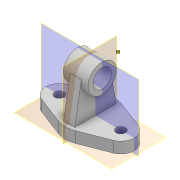
# Autodesk Inventor part: 6.2_DATE11_1
Saved by Autodesk Inventor 2017 (Build 210142000, 142)
## iProperties
Created: 2018-11-01
Part Number: 6.2_DATE11_1
Material: Generic
Document SubType Name: Modeling
Designer: jacob
Density: 1 g/cm^3
Appearance: Default
Mass: 222.641 g
Surface Area: 395.923 cm^2
Volume: 222.641 cm^3
Author: jacob
Autodesk Inventor part; units mm, degrees
sketch "Sketch1" plane through (0, 0, 0) normal (0, 0, 1) x (1, 0, 0)
  circle A0 centre (-49.8513, 0) radius 7.5
  circle A1 centre (50.2519, 0) radius 7.5
  line L0 (-57.7949, 20.5158) -> (-14.443, 37.3015)
  arc A2 (-57.7949, 20.5158) -> (-57.7949, -20.5158) centre (-49.8513, 0) ccw
  arc A3 (58.1322, -20.5402) -> (58.1322, 20.5402) centre (50.2519, 0) ccw
  line L1 (14.3278, 37.3459) -> (58.1322, 20.5402)
  line L2 (58.1322, -20.5402) -> (14.3278, -37.3459)
  line L3 (-57.7949, -20.5158) -> (-14.443, -37.3015)
  arc A4 (-14.443, -37.3015) -> (14.3278, -37.3459) centre (0, 0) ccw
  arc A5 (14.3278, 37.3459) -> (-14.443, 37.3015) centre (0, 0) ccw
  dimension "d19" = 15
  dimension "d20" = 15
  dimension "d45" = 44
  dimension "d46" = 44
  dimension "d47" = 0
  dimension "d48" = 0
  constraints: 8 end point, 8 point on circle, 8 tangent, 6 centre point, 3 coincident
  measures "d19" diameter of A0
  measures "d20" diameter of A1
  measures "d45" diameter of A2
  measures "d46" diameter of A3
  measures "d47" vertical distance of point (0, 0) A0.centre
  measures "d48" vertical distance of point (0, 0) A1.centre
sketch "Sketch2" plane through (0, 0, 0) normal (1, 0, 0) x (0, 1, 0)
  line L0 (-20.5849, 0) -> (20.5849, 0) projected
  line L1 (20.5849, 0) -> (20.5849, 18) projected
  line L2 (-20.5849, 18) -> (-20.5849, 18) projected
  line L3 (-20.5849, 0) -> (-20.5849, 18) projected
  line L4 (-20.5849, 18) -> (-20.5849, 18) projected
  line L5 (-33.5, 18) -> (33.5, 18)
  line L6 (33.5, 18) -> (22.6557, 79.9649)
  line L7 (-22.6557, 79.9649) -> (-33.5, 18)
  circle A0 centre (0, 76) radius 23
  circle A1 centre (0, 76) radius 15
  point P0 (0, 0)
  dimension "d23" = 67
  dimension "d25" = 0
  dimension "d27" = 33.5
  dimension "d37" = 30
  dimension "d38" = 46
  dimension "d39" = 58
  constraints: 6 end point, 2 centre point, 2 point on circle, 2 tangent, 1 coincident, 1 horizontal
  measures "d23" distance of L5.start L5.end
  measures "d25" distance between parallel lines of L2 L5
  measures "d27" horizontal distance of L5.end point (0, 0)
  measures "d37" diameter of A1
  measures "d38" diameter of A0
  measures "d39" distance from line of L5 A0.centre
extrude "Extrusion5" add sketch "Sketch2" along normal mid plane 18 contours L5 L7 A0 L6
extrude "Extrusion6" add sketch "Sketch2" along normal mid plane 40 contours A0
extrude "Extrusion7" add sketch "Sketch1" along normal blind 18
body "Solid1"
